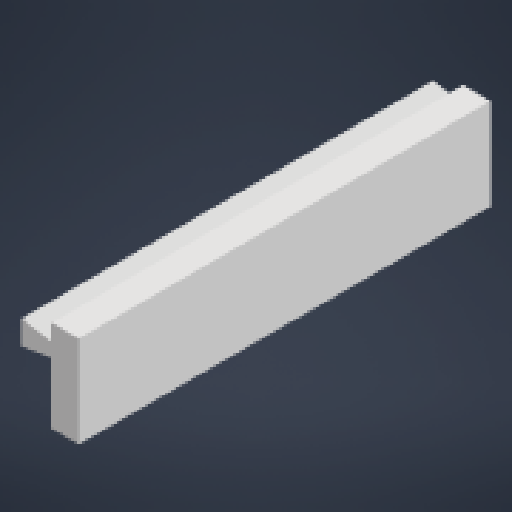
# Autodesk Inventor part: Rack Gripper
Saved by Autodesk Inventor 2026.1 (Build 301233000, 233)
## iProperties
Created: 2025-11-07
Part Number: Rack Gripper
Material: Generic
Document SubType Name: Modeling
Designer: brian
Density: 1 g/cm^3
Appearance: Default
Mass: 1.65338 g
Surface Area: 15.9743 cm^2
Volume: 1.65338 cm^3
Author: brian
Autodesk Inventor part; units mm, degrees
ref_plane "YZ Plane" through (0, 0, 0) normal (1, 0, 0) x (0, 1, 0)
ref_plane "XZ Plane" through (0, 0, 0) normal (0, 1, 0) x (-1, 0, 0)
ref_plane "Work Plane2" through (46.8486, 38.2651, 40.1765) normal (0, 0, 1) x (0, 1, 0)
sketch "Sketch2" plane through (46.8486, 38.2651, 40.1765) normal (0, 0, 1) x (0, 1, 0)
  line L0 (-3.3829, 0) -> (-4, 3.5) projected
  line L1 (-1.6171, 0) -> (-3.3829, 0) projected
  line L2 (-1, 3.5) -> (-1.6171, 0) projected
  line L3 (-4, 3.5) -> (-1, 3.5) projected
  line L4 (-3.8632, 3.3) -> (-3.2813, 0)
  line L5 (-1.8202, 0) -> (-1.2384, 3.3)
  line L6 (-1.2384, 3.3) -> (-3.8632, 3.3)
  line L7 (-1.8202, 0) -> (-1.6171, 0)
  line L8 (0, 0) -> (0, -3)
  line L9 (-3.2813, 0) -> (-3.3829, 0)
  line L10 (-3.3829, 0) -> (-4, 3.5) projected
  line L11 (-4, 3.5) -> (-1, 3.5) projected
  line L12 (-1, 3.5) -> (-1.6171, 0) projected
  line L13 (0, 0) -> (-1.6171, 0) projected
  line L14 (0, 15) -> (0, 0) projected
  line L15 (0, 15) -> (-5, 15) projected
  line L16 (-5, 0) -> (-5, 15) projected
  line L17 (-3.3829, 0) -> (-5, 0) projected
  line L18 (-5, 0) -> (-5, -3)
  line L19 (-5, -3) -> (0, -3)
  line L20 (0, 0) -> (-1.8202, 0)
  line L21 (-3.2813, 0) -> (-5, 0)
  point P0 (-38.2651, 46.8486)
  dimension "d0" = 0.1
  dimension "d1" = 0.2
  dimension "d2" = 3
  dimension "d9" = 90
  constraints: 20 end point, 4 point on line, 3 perpendicular, 2 horizontal, 1 vertical, 1 other
  measures "d0" distance between parallel lines of L0 L4
  measures "d1" distance between parallel lines of L2 L5
  measures "d2" distance of L8.start L8.end
  measures "d9" angle of L14 L9
extrude "Extrusion1" add sketch "Sketch2" against normal blind 45 contours L1 L13 L8 L19 L18 L17 | L4 L6 L5 L1
sketch "Sketch6" plane through (46.8486, 33.2651, 40.1765) normal (0, -1, 0) x (1, 0, 0)
  line L0 (0, 0) -> (0, -45) projected
  line L1 (0, -45) -> (3, -45) projected
  line L2 (0, 0) -> (3, 0)
  line L3 (3, 0) -> (3, -45)
  line L4 (3, -45) -> (0, -45)
  line L5 (0, -45) -> (0, 0)
  point P0 (-46.8486, -40.1765)
  constraints: 8 end point, 2 parallel, 1 horizontal, 1 perpendicular
extrude "Extrusion2" add sketch "Sketch6" along normal blind 5
body "Solid1"
